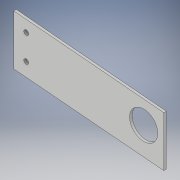
# Autodesk Inventor part: CAR_050_Sweeper Bar arms
Saved by Autodesk Inventor 2018 (Build 220112000, 112)
## iProperties
Created: 2020-02-16
Part Number: CAR_050_Sweeper Bar arms
Material: Generic
Document SubType Name: Modeling
Designer: jd2
Density: 1 g/cm^3
Appearance: Default
Author: jd2
Autodesk Inventor part; units mm, degrees
ref_plane "YZ Plane" through (0, 0, 0) normal (1, 0, 0) x (0, 1, 0)
ref_plane "XZ Plane" through (0, 0, 0) normal (0, 1, 0) x (-1, 0, 0)
ref_plane "XY Plane" through (0, 0, 0) normal (0, 0, 1) x (1, 0, 0)
sketch "Sketch1" plane through (0, 0, 0) normal (0, 0, 1) x (1, 0, 0)
  line L0 (0, 0) -> (151.8201, -13.2825)
  line L1 (151.8201, -13.2825) -> (151.8201, 37.5175)
  line L2 (151.8201, 37.5175) -> (0, 50.8)
  line L3 (0, 50.8) -> (0, 0)
  dimension "d0" = 50.8
  dimension "d1" = 50.8
  dimension "d2" = 85
  dimension "d3" = 152.4
  constraints: 8 end point, 1 parallel, 1 vertical
  measures "d0" distance of L0.end L1.end
  measures "d1" distance of L2.end L0.start
  measures "d2" angle of L2 L3
  measures "d3" distance of L1.end L2.end
extrude "Extrusion1" add sketch "Sketch1" along normal blind 2.54
hole "Hole1" at (131.5001, 16.3479, 2.54) direction (0, 0, -1) diameter 28.575 end through all
sketch "Sketch2" plane through (0, 0, 0) normal (0, 0, -1) x (-1, 0, 0)
  line L0 (0, 0) -> (-151.8201, -13.2825) projected
  line L1 (0, 0) -> (-33.0355, 0)
  line L2 (0, 50.8) -> (0, 0) projected
  point P0 (-12.7, 38.1)
  point P1 (-12.7, 12.7)
  dimension "d15" = 12.7
  dimension "d16" = 38.1
  dimension "d17" = 12.7
  dimension "d18" = 12.7
  constraints: 2 end point, 1 horizontal
  measures "d15" distance from line of L1 point (-12.7, 12.7)
  measures "d16" distance from line of L1 point (-12.7, 38.1)
  measures "d17" distance from line of L2 point (-12.7, 38.1)
  measures "d18" distance from line of L2 point (-12.7, 12.7)
hole "Hole2" at (12.7, 38.1, 0) at (12.7, 12.7, 0) direction (0, 0, 1) diameter 4.8514 end through all
body "Solid1"
